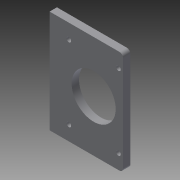
# Autodesk Inventor part: bearing faceplate
Saved by Autodesk Inventor 2013 (Build 170138000, 138)
## iProperties
Created: 2013-01-20
Part Number: bearing faceplate
Material: Generic
Document SubType Name: Sheet Metal
Designer: Arpan
Density: 1 g/cm^3
Sheet Metal Rule: Default
Author: Arpan
Autodesk Inventor part; units mm, degrees
ref_plane "YZ Plane" through (0, 0, 0) normal (1, 0, 0) x (0, 1, 0)
ref_plane "XZ Plane" through (0, 0, 0) normal (0, 1, 0) x (-1, 0, 0)
ref_plane "XY Plane" through (0, 0, 0) normal (0, 0, 1) x (1, 0, 0)
sketch "Sketch1" plane through (0, 0, 0) normal (0, 0, 1) x (1, 0, 0)
  line L0 (-3.175, 0) -> (-63.5, 0)
  line L1 (0, 3.175) -> (0, 85.725)
  line L2 (-3.175, 88.9) -> (-63.5, 88.9)
  line L3 (-63.5, 88.9) -> (-63.5, 0)
  circle A0 centre (-3.9688, 76.2) radius 1.9844
  circle A1 centre (-3.9688, 12.7) radius 1.9844
  circle A2 centre (-46.8313, 12.7) radius 1.9812
  circle A3 centre (-46.8313, 76.2) radius 1.9812
  arc A4 (0, 85.725) -> (-3.175, 88.9) centre (-3.175, 85.725) ccw
  arc A5 (-3.175, 0) -> (0, 3.175) centre (-3.175, 3.175) ccw
  point P0 (0, 0)
  point P1 (0, 88.9)
  dimension "d0" = 63.5
  dimension "d1" = 88.9
  dimension "d2" = 3.9688
  dimension "d3" = 3.9688
  dimension "d4" = 3.9624
  dimension "d5" = 3.9624
  dimension "d6" = 12.7
  dimension "d7" = 12.7
  dimension "d8" = 12.7
  dimension "d9" = 3.9688
  dimension "d10" = 3.9688
  dimension "d11" = 16.6687
  dimension "d12" = 12.7
  dimension "d13" = 16.6687
  dimension "d19" = 3.175
  measures "d0" distance of point (0, 0) L0.end
  measures "d1" distance of point (0, 0) point (0, 88.9)
  measures "d2" diameter of A0
  measures "d3" diameter of A1
  measures "d4" diameter of A2
  measures "d5" diameter of A3
  measures "d6" distance from line of A1.centre L0
  measures "d7" distance from line of L2 A0.centre
  measures "d8" distance from line of L2 A3.centre
  measures "d9" distance from line of L1 A0.centre
  measures "d10" distance from line of L1 A1.centre
  measures "d11" distance from line of L3 A2.centre
  measures "d12" distance from line of L0 A2.centre
  measures "d13" distance from line of L3 A3.centre
  measures "d19" radius of A4
extrude "Plate1" add sketch "Sketch1" along normal blind 6.35
sketch "Sketch2" plane through (0, 0, 6.35) normal (0, 0, 1) x (1, 0, 0)
  line L0 (0, 85.725) -> (0, 3.175) projected
  line L1 (-63.5, 88.9) -> (-3.175, 88.9) projected
  line L2 (0, 44.45) -> (-25.4, 44.45)
  circle A0 centre (-25.4, 44.45) radius 19.05
  point P0 (0, 0)
  point P1 (0, 88.9)
  dimension "d15" = 25.4
  dimension "d16" = 38.1
  constraints: 2 end point, 1 centre point, 1 coincident, 1 midpoint, 1 parallel
  measures "d15" distance of L2.start L2.end
  measures "d16" diameter of A0
extrude "Cut1" cut sketch "Sketch2" against normal blind 6.35
equation "\"d17\" = Thickness"
equation "\"BendRadius\" = Thickness"
equation "\"BendReliefWidth\" = Thickness"
equation "\"BendReliefDepth\" = 0.5 * Thickness"
equation "\"CornerReliefSize\" = 4 * Thickness"
equation "\"MinimumRemnant\" = 2 * Thickness"
equation "\"TransitionRadius\" = BendRadius"
equation "\"JacobiRadiusSize\" = BendRadius"
equation "\"GapSize\" = Thickness"
equation "\"d14\" = BendRadius"
equation "\"Thickness\" = 6.35"
body "Solid1"
